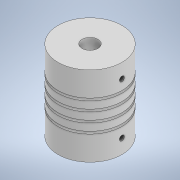
# Autodesk Inventor part: KN_5_8
Saved by Autodesk Inventor 2022 (Build 260153000, 153)
## iProperties
Created: 2022-11-10
Part Number: KN_5_8
Material: Generic
Document SubType Name: Modeling
Designer: nguye
Density: 1 g/cm^3
Appearance: Default
Author: nguye
Autodesk Inventor part; units mm, degrees
ref_plane "XZ Plane" through (0, 0, 0) normal (0, 1, 0) x (-1, 0, 0)
ref_plane "XY Plane" through (0, 0, 0) normal (0, 0, 1) x (1, 0, 0)
sketch "Sketch1" plane through (0, 0, 0) normal (0, 1, 0) x (-1, 0, 0)
  circle A0 centre (0, 0) radius 10
  dimension "d0" = 20
  constraints: 1 centre point, 1 coincident
  measures "d0" diameter of A0
extrude "Extrusion1" add sketch "Sketch1" along normal blind 25
sketch "Sketch2" plane through (0, 25, 0) normal (0, 1, 0) x (1, 0, 0)
  circle A0 centre (0, 0) radius 10 projected
  constraints: 1 coincident
hole "Hole1" at (0, 25, 0) direction (0, -1, 0) diameter 5 depth 10
sketch "Sketch3" plane through (0, 0, 0) normal (0, -1, 0) x (1, 0, 0)
  circle A0 centre (0, 0) radius 10 projected
  constraints: 1 coincident
hole "Hole2" at (0, 0, 0) direction (0, 1, 0) diameter 6.647 depth 10 thread size "M8x1.25" class "6H" standard "ISO Metric profile"
sketch "Sketch4" plane through (0, 0, 0) normal (1, 0, 0) x (0, 1, 0)
  circle A0 centre (17, 10) radius 0.375
  line L0 (0, 10) -> (25, 10) projected
  circle A1 centre (14, 10) radius 0.375
  circle A2 centre (11, 10) radius 0.375
  circle A3 centre (8, 10) radius 0.375
  line L1 (17.375, 10) -> (7.625, 10)
  line L2 (-5, 0) -> (30, 0) projected
  point P0 (0, 0)
  point P1 (8.375, 10)
  point P2 (11.375, 10)
  point P3 (10.625, 10)
  point P4 (14.375, 10)
  point P5 (13.625, 10)
  point P6 (16.625, 10)
  dimension "d21" = 0.75
  dimension "d17" = 8
  dimension "d18" = 3
  dimension "d19" = 3
  dimension "d20" = 3
  constraints: 4 horizontal alignment, 4 point on line, 2 centre point, 2 end point, 1 equal radius, 8 other
  measures "d17" distance of L0.start point (8, 10)
  measures "d18" distance of A2.centre point (8, 10)
  measures "d19" distance of A2.centre A1.centre
  measures "d20" distance of A1.centre point (17, 10)
revolve "Revolution1" cut sketch "Sketch4" angle 360 about axis through (0, -10, 0) along (0, 1, 0) picked at (8.0151, 9.8759) picked at (10.9849, 9.8759) picked at (13.9849, 9.8759) picked at (17.0151, 9.8759) contours A3 L0 | A2 L0 | A1 L0 | A0 L0
ref_plane "Work Plane1" through (-10, 0, 0) normal (1, 0, 0) x (0, 1, 0)
sketch "Sketch5" plane through (-10, 0, 0) normal (1, 0, 0) x (0, 1, 0)
  point P0 (0, 0)
  point P1 (20.5, 0)
  point P2 (4.5, 0)
  dimension "d23" = 16
  dimension "d24" = 4.5
  constraints: 2 horizontal alignment
  measures "d23" distance of point (4.5, 0) point (20.5, 0)
  measures "d24" distance of point (4.5, 0) point (0, 0)
hole "Hole3" at (-10, 20.5, 0) at (-10, 4.5, 0) direction (1, 0, 0) diameter 1.567 end through all thread size "M2x0.4" class "6H" standard "ISO Metric profile"
body "Solid1"
